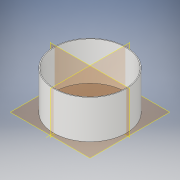
# Autodesk Inventor part: FrisbeeHopperV02
Saved by Autodesk Inventor 2019.4 (Build 234330000, 330)
## iProperties
Created: 2015-07-20
Part Number: FrisbeeHopperV02
Material: PC/ABS Plastic
Document SubType Name: Modeling
Designer: steele
Density: 0.357273 g/cm^3
Appearance: Smooth - White
Mass: 146.454 g
Surface Area: 2639.82 cm^2
Volume: 409.921 cm^3
Author: steele
Autodesk Inventor part; units mm, degrees
sketch "Sketch1" plane through (0, 0, 0) normal (0, 1, 0) x (-1, 0, 0)
  circle A0 centre (0, 0) radius 142.875
  circle A1 centre (0, 0) radius 146.05
  circle A2 centre (0, 0) radius 139.7 construction
  dimension "interiorDiam" = 285.75
  dimension "exteriorDiam" = 292.1
  dimension "frisbeeDiam" = 279.4
  constraints: 3 centre point, 3 coincident
  measures "interiorDiam" diameter of A0
  measures "exteriorDiam" diameter of A1
  measures "frisbeeDiam" diameter of A2
extrude "Extrusion1" add sketch "Sketch1" along normal blind 154.94
body "Solid1"
